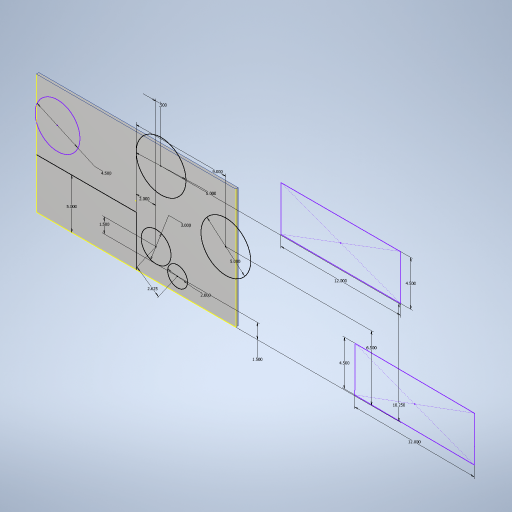
# Autodesk Inventor part: Int1-001
Saved by Autodesk Inventor 2023.4 (Build 274418000, 418)
## iProperties
Created: 2025-01-12
Part Number: Int1-001
Material: Aluminum 6061
Document SubType Name: Modeling
Designer: mavericks
Density: 2.7 g/cm^3
Appearance: Aluminum - Flat
Author: mavericks
Autodesk Inventor part; units mm, degrees
ref_plane "YZ Plane" through (0, 0, 0) normal (1, 0, 0) x (0, 1, 0)
ref_plane "XZ Plane" through (0, 0, 0) normal (0, 1, 0) x (-1, 0, 0)
ref_plane "XY Plane" through (0, 0, 0) normal (0, 0, 1) x (1, 0, 0)
sketch "Sketch1" plane through (0, 0, 0) normal (0, 0, 1) x (1, 0, 0)
  line L0 (-254, -152.4) -> (254, -152.4)
  line L1 (254, -152.4) -> (254, 152.4)
  line L2 (254, 152.4) -> (-254, 152.4)
  line L3 (-254, 152.4) -> (-254, -152.4)
  line L4 (-254, -152.4) -> (254, 152.4) construction
  line L5 (254, -152.4) -> (-254, 152.4) construction
  point P0 (0, 0)
  dimension "d0" = 508
  dimension "d1" = 304.8
  constraints: 12 end point, 2 midpoint, 2 parallel, 1 horizontal, 1 perpendicular
  measures "d0" distance of L2.end L1.end
  measures "d1" distance of L1.end L0.end
extrude "Extrusion1" add sketch "Sketch1" along normal blind 6.35
sketch "Sketch2" plane through (0, 0, 6.35) normal (0, 0, 1) x (1, 0, 0)
  line L0 (-254, 152.4) -> (-254, -152.4) projected
  line L1 (-254, -25.4) -> (0, -25.4)
  line L2 (0, -25.4) -> (0, -152.4)
  line L3 (-254, -152.4) -> (254, -152.4) projected
  line L4 (254, -152.4) -> (254, 152.4) projected
  circle A0 centre (105.517, -114.3) radius 25.4
  circle A1 centre (228.6, 12.7) radius 63.5
  line L5 (369.0504, 224.433) -> (673.8504, 224.433)
  line L6 (673.8504, 224.433) -> (673.8504, 110.133)
  line L7 (673.8504, 110.133) -> (369.0504, 110.133)
  line L8 (369.0504, 110.133) -> (369.0504, 224.433)
  line L9 (369.0504, 224.433) -> (673.8504, 110.133) construction
  line L10 (673.8504, 224.433) -> (369.0504, 110.133) construction
  line L11 (862.0232, -152.4) -> (557.2308, -150.2422)
  line L12 (557.2308, -150.2422) -> (558.04, -35.945)
  line L13 (558.04, -35.945) -> (862.8324, -38.1029)
  line L14 (862.8324, -38.1029) -> (862.0232, -152.4)
  line L15 (862.0232, -152.4) -> (558.04, -35.945) construction
  line L16 (557.2308, -150.2422) -> (862.8324, -38.1029) construction
  circle A2 centre (-200.3882, 65.4535) radius 57.15
  circle A3 centre (50.8, -76.2) radius 38.1
  circle A4 centre (63.5, 107.95) radius 63.5
  point P0 (0, 0)
  point P1 (521.4504, 167.283)
  point P2 (710.0316, -94.1725)
  dimension "d4" = 127
  dimension "d6" = 50.8
  dimension "d7" = 127
  dimension "d9" = 304.8
  dimension "d10" = 114.3
  dimension "d11" = 38.1
  dimension "d12" = 165.1
  dimension "d14" = 304.8
  dimension "d15" = 114.3
  dimension "d16" = 114.3
  dimension "d17" = 76.2
  dimension "d18" = 38.1
  dimension "d19" = 66.675
  dimension "d20" = 127
  dimension "d21" = 260.35
  dimension "d22" = 50.8
  dimension "d23" = 228.6
  dimension "d24" = 12.7
  constraints: 28 end point, 5 centre point, 5 midpoint, 4 parallel, 3 perpendicular, 2 horizontal, 2 point on line, 1 vertical alignment
  measures "d4" distance between parallel lines of L3 L1
  measures "d6" diameter of A0
  measures "d7" diameter of A1
  measures "d9" distance of L6.end L7.end
  measures "d10" distance of L5.end L6.end
  measures "d11" distance from line of L3 A0.centre
  measures "d12" distance from line of A1.centre L3
  measures "d14" distance of L11.start L11.end
  measures "d15" distance of L11.end L12.end
  measures "d16" diameter of A2
  measures "d17" diameter of A3
  measures "d18" vertical distance of A0.centre A3.centre
  measures "d19" distance of A0.centre A3.centre
  measures "d20" diameter of A4
  measures "d21" distance from line of L3 A4.centre
  measures "d22" distance from line of L2 A3.centre
  measures "d23" distance from line of A1.centre L2
  measures "d24" horizontal distance of A3.centre A4.centre
body "Solid1"
